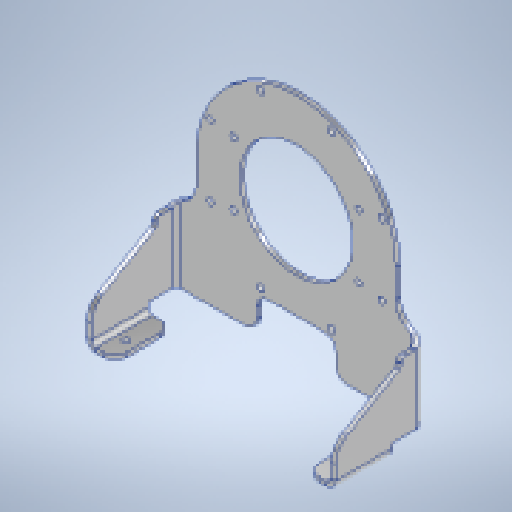
# Autodesk Inventor part: basefixplate2_forR6
Saved by Autodesk Inventor 2024.3 (Build 283343010, 343A)
## iProperties
Created: 2025-05-24
Part Number: basefixplate2_forR6
Material: アルミニウム 6061
Document SubType Name: Sheet Metal
Designer: kshau
Density: 2.7 g/cm^3
Sheet Metal Rule: Default
Appearance: アルミニウム - フラット
Mass: 59.4336 g
Surface Area: 238.01 cm^2
Volume: 22.0124 cm^3
Flat Pattern Width: 11.455 cm
Flat Pattern Length: 18.2 cm
Flat Pattern Area: 208.481 cm^2
Sheet Metal Width: 114.550 mm
Sheet Metal Length: 182.000 mm
Sheet Metal Area: 20848.100 mm^2
Author: kshau
Autodesk Inventor part; units mm, degrees
ref_plane "YZ Plane" through (0, 0, 0) normal (1, 0, 0) x (0, 1, 0)
ref_plane "XZ Plane" through (0, 0, 0) normal (0, 1, 0) x (-1, 0, 0)
ref_plane "XY Plane" through (0, 0, 0) normal (0, 0, 1) x (1, 0, 0)
sketch "スケッチ1" plane through (0, 0, 0) normal (0, 0, 1) x (1, 0, 0)
  circle A0 centre (0, 0) radius 44
  line L0 (0, -55.55) -> (0, 0)
  line L1 (0, -55.55) -> (44, -55.55)
  line L2 (44, 0) -> (44, -55.55)
  line L3 (0, -55.55) -> (-44, -55.55)
  line L4 (-44, 0) -> (-44, -55.55)
  circle A1 centre (0, 0) radius 25
  point P0 (0, -44)
  point P1 (-44, 0)
  dimension "d0" = 88
  dimension "d4" = 50
  dimension "d170" = 55.55
  measures "d0" diameter of A0
  measures "d4" diameter of A1
  measures "d170" distance from line of L1 point (0, 0)
extrude "プレート1" add sketch "スケッチ1" along normal blind 2
sketch "スケッチ2" plane through (0, 0, 2) normal (0, 0, 1) x (1, 0, 0)
  line L0 (-44, 0) -> (-44, -55.55)
  line L1 (-44, -55.55) -> (-91, -55.55)
  line L2 (-91, -55.55) -> (-44, -55.55)
  line L3 (-44, -55.55) -> (-44, -45.55)
  line L4 (-44, -45.55) -> (-91, -45.55)
  line L5 (-91, -45.55) -> (-91, -55.55)
  line L6 (-91, -45.55) -> (-44, -18)
  line L7 (-91, -55.55) -> (-66, -55.55)
  line L8 (-66, -55.55) -> (-66, -70.55)
  line L9 (-66, -70.55) -> (-91, -70.55)
  line L10 (-91, -70.55) -> (-91, -55.55)
  line L11 (0, 0) -> (0, -55.55)
  line L12 (-44, -55.55) -> (44, -55.55)
  line L13 (44, 0) -> (44, -55.55)
  line L14 (44, -55.55) -> (91, -55.55)
  line L15 (44, -45.55) -> (91, -45.55)
  line L16 (91, -45.55) -> (91, -55.55)
  line L17 (91, -45.55) -> (44, -18)
  line L18 (66, -55.55) -> (66, -70.55)
  line L19 (66, -70.55) -> (91, -70.55)
  line L20 (91, -70.55) -> (91, -55.55)
  line L21 (-51, -55.55) -> (-51, -22.1032)
  line L22 (51, -55.55) -> (51, -22.1032)
  line L23 (-91, -59.55) -> (-66, -59.55)
  line L24 (91, -59.55) -> (66, -59.55)
  line L25 (-55.9777, -25.021) -> (-62, -25.021)
  line L26 (-62, -25.021) -> (-62, -55.55)
  line L27 (-62, -55.55) -> (-55.9777, -55.55)
  line L28 (-55.9777, -55.55) -> (-55.9777, -25.021)
  line L29 (55.9777, -25.021) -> (62, -25.021)
  line L30 (62, -25.021) -> (62, -55.55)
  line L31 (55.9777, -55.55) -> (55.9777, -25.021)
  point P0 (66, -55.55)
  point P1 (-62, -28.5511)
  point P2 (55.9777, -25.021)
  point P3 (62, -28.5511)
  dimension "d6" = 10
  dimension "d7" = 18
  dimension "d9" = 15
  dimension "d132" = 51
  dimension "d157" = 25
  dimension "d160" = 40
  dimension "d163" = 4
  dimension "d164" = 91
  dimension "d167" = 29
  dimension "d168" = 25.021
  measures "d6" distance of L4.end L1.end
  measures "d7" distance of L0.start L6.end
  measures "d9" distance of L9.end L1.end
  measures "d132" distance between parallel lines of L11 L21
  measures "d157" distance between parallel lines of L10 L8
  measures "d160" distance between parallel lines of L21 L5
  measures "d163" distance between parallel lines of L1 L23
  measures "d164" distance between parallel lines of L11 L10
  measures "d167" distance between parallel lines of L5 L26
  measures "d168" distance from line of L11.start L25
sheet face with bend "面2" sketch "スケッチ2" thickness 2 toward (0, 0, -1) bend radius 2
bend "曲げ1"
sketch "スケッチ3" plane through (0, 0, 2) normal (0, 0, 1) x (1, 0, 0)
  line L0 (-66, -55.55) -> (66, -55.55) projected
  line L1 (-51, -55.55) -> (-51, -22.1032)
  line L2 (-44, -18) -> (-91, -45.55) projected
  line L3 (-66, -70.55) -> (-66, -55.55) projected
  line L4 (0, 0) -> (0, -55.55)
  dimension "d158" = 51
  constraints: 4 end point, 2 point on line, 1 midpoint, 1 vertical
  measures "d158" distance between parallel lines of L4 L1
fold "折り曲げ1" angle 90 bend radius 2 thickness 2 k factor 0.44 line from (-51, -55.55, 2) to (-51, -22.1032, 2) line at bend start moving side (-1, 0, 0) folds toward (0, 0, 1)
sketch "スケッチ4" plane through (0, 0, 2) normal (0, 0, 1) x (1, 0, 0)
  line L0 (91, -45.55) -> (44, -18) projected
  line L1 (51, -22.1032) -> (51, -55.55)
  line L2 (-51, -55.55) -> (66, -55.55) projected
  line L3 (66, -55.55) -> (66, -70.55) projected
  line L4 (0, 0) -> (0, -55.55)
  dimension "d159" = 51
  constraints: 4 end point, 3 point on line, 1 perpendicular, 1 vertical
  measures "d159" distance between parallel lines of L4 L1
fold "折り曲げ2" angle 90 bend radius 2 thickness 2 k factor 0.44 line from (51, -22.1032, 2) to (51, -55.55, 2) line at bend start moving side (1, 0, 0) folds toward (0, 0, 1)
sketch "スケッチ10" plane through (0, 0, 2) normal (0, 0, 1) x (1, 0, 0)
  circle A0 centre (0, 0) radius 31
  line L0 (0, 0) -> (0, 31)
  line L1 (0, 0) -> (-27.6333, 14.05)
  line L2 (0, 0) -> (-31, 0)
  point P0 (27.6333, 14.05)
  point P1 (-27.6333, -14.05)
  point P2 (27.6333, -14.05)
  dimension "d60" = 62
  dimension "d89" = 14.05
  constraints: 6 end point, 3 point on circle, 3 symmetric about line, 2 coincident, 1 centre point, 1 horizontal, 1 vertical
  measures "d60" diameter of A0
  measures "d89" distance from line of L2 point (-27.633, 14.05)
hole "穴1" at (-27.6333, 14.05, 2) at (-27.6333, -14.05, 2) at (27.6333, -14.05, 2) at (27.6333, 14.05, 2) direction (0, 0, -1) diameter 3 end through all
sketch "スケッチ14" plane through (0, 0, 2) normal (0, 0, 1) x (1, 0, 0)
  circle A0 centre (0, 0) radius 41
  line L0 (0, 0) -> (-15.69, 37.8791)
  line L1 (0, 0) -> (0, 41)
  point P0 (-37.8791, 15.69)
  point P1 (-37.8791, -15.69)
  point P2 (-15.69, -37.8791)
  point P3 (15.69, -37.8791)
  point P4 (37.8791, -15.69)
  point P5 (37.8791, 15.69)
  point P6 (15.69, 37.8791)
  dimension "d90" = 82
  dimension "d91" = 22.5
  dimension "d94" = 360
  constraints: 4 end point, 2 coincident, 2 point on circle, 1 centre point, 1 vertical, 9 other
  measures "d90" diameter of A0
  measures "d91" angle of L1 L0
hole "穴3" at (-15.69, 37.8791, 2) at (-37.8791, 15.69, 2) at (-37.8791, -15.69, 2) at (-15.69, -37.8791, 2) at (15.69, -37.8791, 2) at (37.8791, -15.69, 2) at (37.8791, 15.69, 2) at (15.69, 37.8791, 2) direction (0, 0, -1) diameter 3 end through all
sketch "スケッチ17" plane through (0, 0, 2) normal (0, 0, 1) x (1, 0, 0)
  line L0 (-51, -55.55) -> (51, -55.55) projected
  line L1 (0, -55.55) -> (17.5, -55.55)
  line L2 (17.5, -55.55) -> (17.5, -40.55)
  line L3 (17.5, -40.55) -> (0, -40.55)
  line L4 (0, -40.55) -> (0, -55.55)
  line L5 (-17.5, -55.55) -> (-17.5, -40.55)
  line L6 (-17.5, -40.55) -> (0, -40.55)
  point P0 (0, 0)
  dimension "d114" = 15
  dimension "d115" = 17.5
  constraints: 12 end point, 2 parallel, 2 symmetric about line, 1 horizontal, 1 midpoint, 1 perpendicular
  measures "d114" distance of L1.end L2.end
  measures "d115" distance of L2.end L3.end
extrude "押し出し5" cut sketch "スケッチ17" against normal blind 4
sketch "スケッチ19" plane through (-53, -70.55, 39.4761) normal (1, 0, 0) x (0, 0, -1)
  line L0 (25, 0) -> (25, 15) projected
  line L1 (25, 13) -> (0, 13)
  line L2 (0, 25) -> (0, 0) projected
  line L3 (0, 0) -> (25, 0) projected
  line L4 (25, 15) -> (35.4761, 15) projected
  point P0 (39.4761, 70.55)
  dimension "d161" = 2
  constraints: 2 end point, 2 point on line, 1 horizontal
  measures "d161" distance between parallel lines of L4 L1
fold "折り曲げ7" angle 90 bend radius 2 thickness 2 k factor 0.44 line from (-53, -57.55, 14.4761) to (-53, -57.55, 39.4761) line at bend start moving side (0, -1, 0) folds toward (1, 0, 0)
sketch "スケッチ20" plane through (53, -70.55, 39.4761) normal (-1, 0, 0) x (0, 0, 1)
  line L0 (-25, 15) -> (-25, 0) projected
  line L1 (-25, 13) -> (0, 13)
  line L2 (0, 0) -> (0, 25) projected
  line L3 (-25, 0) -> (0, 0) projected
  line L4 (-35.4761, 15) -> (-25, 15) projected
  point P0 (-39.4761, 70.55)
  dimension "d162" = 2
  constraints: 2 end point, 2 point on line, 1 horizontal
  measures "d162" distance between parallel lines of L4 L1
fold "折り曲げ8" angle 90 bend radius 2 thickness 2 k factor 0.44 line from (53, -57.55, 14.4761) to (53, -57.55, 39.4761) line at bend start moving side (0, -1, 0) folds toward (-1, 0, 0)
sketch "スケッチ21" plane through (42.5239, -61.55, 39.4761) normal (0, -1, 0) x (1, 0, 0)
  line L0 (-42.5239, -39.4761) -> (-42.5239, -66.4761)
  circle A0 centre (-42.5239, -66.4761) radius 74
  point P0 (-89.5239, -9.3184)
  point P1 (4.4761, -9.3184)
  dimension "d148" = 148
  dimension "d147" = 27
  dimension "d149" = 47
  constraints: 2 end point, 1 coincident, 1 symmetric about line, 1 vertical, 3 other
  measures "d147" distance of L0.start L0.end
  measures "d149" distance from line of L0 point (-89.524, -9.318)
hole "穴6" at (-47, -61.55, 30.1577) at (47, -61.55, 30.1577) direction (0, 1, 0) diameter 3 end through all
fillet "フィレット5" radius 5 8 edges at (-17.5, -55.55, 1) (-17.5, -40.55, 1) (17.5, -40.55, 1) (17.5, -55.55, 1) (-42.5239, -60.55, 39.4761) (-42.5239, -60.55, 14.4761) (42.5239, -60.55, 39.4761) (42.5239, -60.55, 14.4761)
fillet "フィレット6" radius 10 4 edges at (-44, -18, 1) (44, -18, 1) (-54, -45.55, 39.4761) (54, -45.55, 39.4761)
fillet "フィレット7" radius 2 4 edges at (54, -28.5511, 10.4761) (54, -25.021, 10.4761) (-54, -28.5511, 10.4761) (-54, -25.021, 10.4761)
fillet "フィレット8" radius 2 2 edges at (-54, -55.55, 14.4761) (54, -55.55, 14.4761)
equation "\"d149\" = Almiwidth1"
equation "\"d132\" = Almiwidth2"
equation "\"d164\" = Almiwidth3"
equation "\"d158\" = Almiwidth2"
equation "\"d5\" = Thickness"
equation "\"d17\" = BendReliefWidth"
equation "\"d18\" = BendReliefDepth"
equation "\"d19\" = MinimumRemnant"
equation "\"d20\" = TransitionRadius"
equation "\"d22\" = BendRadius"
equation "\"d159\" = Almiwidth2"
equation "\"d25\" = BendReliefWidth"
equation "\"d26\" = BendReliefDepth"
equation "\"d27\" = MinimumRemnant"
equation "\"d28\" = TransitionRadius"
equation "\"d30\" = BendRadius"
equation "\"d71\" = Thickness"
equation "\"d101\" = Thickness"
equation "\"d134\" = BendReliefWidth"
equation "\"d135\" = BendReliefDepth"
equation "\"d136\" = MinimumRemnant"
equation "\"d137\" = TransitionRadius"
equation "\"d139\" = BendRadius"
equation "\"d141\" = BendReliefWidth"
equation "\"d142\" = BendReliefDepth"
equation "\"d143\" = MinimumRemnant"
equation "\"d144\" = TransitionRadius"
equation "\"d146\" = BendRadius"
equation "\"d148\" = Radius1"
equation "\"d147\" = 0.5 * R06Thick + 0.5 * Thick1"
equation "\"d11\" = BendRadius"
equation "\"d12\" = BendReliefWidth"
equation "\"d14\" = MinimumRemnant"
equation "\"d13\" = BendReliefDepth"
equation "\"d15\" = TransitionRadius"
equation "\"Thickness\" = Almithick1"
equation "\"BendRadius\" = Thickness"
equation "\"BendReliefWidth\" = Thickness"
equation "\"BendReliefDepth\" = 0.5 * Thickness"
equation "\"CornerReliefSize\" = 4 * Thickness"
equation "\"MinimumRemnant\" = 2 * Thickness"
equation "\"TransitionRadius\" = BendRadius"
equation "\"JacobiRadiusSize\" = BendRadius"
equation "\"GapSize\" = Thickness"
equation "\"Almiwidth2\" = 51"
equation "\"Almiwidth3\" = 91"
equation "\"Radius1\" = 148"
equation "\"R06Thick\" = 49"
equation "\"Thick1\" = 5"
equation "\"Almithick1\" = 2"
equation "\"Almiwidth1\" = 47"
